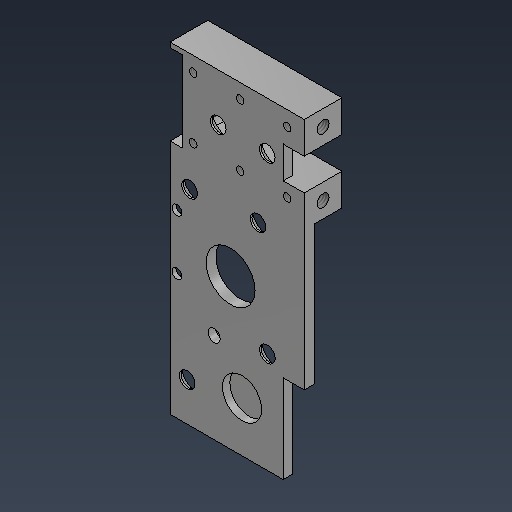
# Autodesk Inventor part: LeftGearboxCoverr
Saved by Autodesk Inventor 2026.2 (Build 302298010, 298A)
## iProperties
Created: 2026-04-13
Part Number: LeftGearboxCoverr
Material: Nylon 6/6
Document SubType Name: Modeling
Designer: szymo
Density: 1.13 g/cm^3
Appearance: Nylon 6(1)
Mass: 4.78265 g
Surface Area: 44.1112 cm^2
Volume: 4.23243 cm^3
Author: szymo
Autodesk Inventor part; units mm, degrees
ref_plane "YZ Plane" through (0, 0, 0) normal (1, 0, 0) x (0, 1, 0)
ref_plane "XZ Plane" through (0, 0, 0) normal (0, 1, 0) x (-1, 0, 0)
ref_plane "XY Plane" through (0, 0, 0) normal (0, 0, 1) x (1, 0, 0)
sketch "Sketch1" plane through (0, 0, 0) normal (0, 0, 1) x (1, 0, 0)
  circle A0 centre (14.7, -55.6371) radius 14.7 construction
  circle A1 centre (12.35, -35.2722) radius 5
  circle A2 centre (14.7, -14.7) radius 14.7 construction
  line L0 (23.1, -65.8371) -> (0, -65.8371)
  line L1 (0, -65.8371) -> (0, 0)
  line L2 (0, 0) -> (27.4, 0)
  line L3 (27.4, 0) -> (27.4, -19.5)
  line L4 (2.5, -1) -> (2.5, -9.4261)
  line L5 (2.5, -1) -> (1, -1)
  line L6 (1, -1) -> (1, -1)
  line L7 (1, -1) -> (0, -1)
  line L8 (2.5, -9.4261) -> (2.5, -17.5)
  line L9 (2.5, -17.5) -> (1, -17.5)
  line L10 (1, -17.5) -> (1, -17.5)
  line L11 (1, -17.5) -> (0, -17.5)
  line L12 (7.8075, -6.5) -> (27.4, -6.5)
  line L13 (7.8075, -6.5) -> (2.5, -6.5)
  line L14 (2.5, -13) -> (27.4, -13)
  line L15 (0, -19.5) -> (27.4, -19.5)
  circle A3 centre (14.7, -55.6371) radius 4
  circle A4 centre (9.002, -47.4193) radius 1.25
  line L16 (23.1, -13) -> (23.1, -6.5)
  circle A5 centre (14.7, -55.6371) radius 14.7 projected
  circle A6 centre (14.7, -55.6371) radius 14 projected
  line L17 (6.8877, -8.4575) -> (4.7029, -7.1961) projected
  arc A7 (4.7029, -7.1961) -> (3.2029, -9.7942) centre (14.7, -14.7) ccw projected
  line L18 (3.2029, -9.7942) -> (5.3877, -11.0556) projected
  arc A8 (6.8877, -8.4575) -> (5.3877, -11.0556) centre (14.7, -14.7) ccw projected
  arc A9 (24.6971, -22.2039) -> (26.1971, -19.6058) centre (14.7, -14.7) ccw projected
  line L19 (26.1971, -19.6058) -> (24.0123, -18.3444) projected
  arc A10 (22.5123, -20.9425) -> (24.0123, -18.3444) centre (14.7, -14.7) ccw projected
  line L20 (22.5123, -20.9425) -> (24.6971, -22.2039) projected
  circle A11 centre (14.7, -14.7) radius 5 projected
  circle A12 centre (14.7, -14.7) radius 14 projected
  circle A13 centre (14.7, -14.7) radius 14.7 projected
  circle A14 centre (14.7, -14.7) radius 14 projected
  circle A15 centre (12.35, -35.2722) radius 5 projected
  circle A16 centre (12.35, -35.2722) radius 5.4 projected
  line L21 (1.5, -1) -> (1.5, -17) projected
  line L22 (2.5, -1) -> (1.5, -1) projected
  line L23 (2.5, -17) -> (2.5, -1) projected
  line L24 (2.5, -17) -> (1.5, -17) projected
  circle A17 centre (9.002, -47.4193) radius 1.25 projected
  arc A18 (10.0798, -44.7809) -> (10.0692, -43.3571) centre (6.4391, -44.096) ccw projected
  arc A19 (10.4149, -44.9442) -> (10.0798, -44.7809) centre (9.002, -47.4193) ccw projected
  arc A20 (11.5425, -44.0747) -> (10.4149, -44.9442) centre (13.1986, -47.3885) ccw projected
  arc A21 (11.9573, -44.4349) -> (11.5425, -44.0747) centre (9.002, -47.4193) ccw projected
  arc A22 (11.2545, -45.6733) -> (11.9573, -44.4349) centre (8.4441, -43.2598) ccw projected
  arc A23 (11.4632, -45.9822) -> (11.2545, -45.6733) centre (9.002, -47.4193) ccw projected
  arc A24 (12.8744, -45.7931) -> (11.4632, -45.9822) centre (12.6518, -49.4909) ccw projected
  arc A25 (13.0535, -46.3124) -> (12.8744, -45.7931) centre (9.002, -47.4193) ccw projected
  arc A26 (11.8257, -47.0335) -> (13.0535, -46.3124) centre (10.5986, -43.5381) ccw projected
  arc A27 (11.8519, -47.4053) -> (11.8257, -47.0335) centre (9.002, -47.4193) ccw projected
  arc A28 (13.1687, -47.9471) -> (11.8519, -47.4053) centre (11.1269, -51.0383) ccw projected
  arc A29 (13.0641, -48.4865) -> (13.1687, -47.9471) centre (9.002, -47.4193) ccw projected
  arc A30 (11.6403, -48.497) -> (13.0641, -48.4865) centre (12.3253, -44.8564) ccw projected
  arc A31 (11.4771, -48.8322) -> (11.6403, -48.497) centre (9.002, -47.4193) ccw projected
  arc A32 (12.3465, -49.9598) -> (11.4771, -48.8322) centre (9.0327, -51.6159) ccw projected
  arc A33 (11.9863, -50.3746) -> (12.3465, -49.9598) centre (9.002, -47.4193) ccw projected
  arc A34 (10.748, -49.6718) -> (11.9863, -50.3746) centre (13.1615, -46.8614) ccw projected
  arc A35 (10.439, -49.8804) -> (10.748, -49.6718) centre (9.002, -47.4193) ccw projected
  arc A36 (10.6282, -51.2917) -> (10.439, -49.8804) centre (6.9303, -51.069) ccw projected
  arc A37 (10.1088, -51.4708) -> (10.6282, -51.2917) centre (9.002, -47.4193) ccw projected
  arc A38 (9.3878, -50.243) -> (10.1088, -51.4708) centre (12.8832, -49.0159) ccw projected
  arc A39 (9.0159, -50.2692) -> (9.3878, -50.243) centre (9.002, -47.4193) ccw projected
  arc A40 (8.4741, -51.586) -> (9.0159, -50.2692) centre (5.383, -49.5442) ccw projected
  arc A41 (7.9347, -51.4814) -> (8.4741, -51.586) centre (9.002, -47.4193) ccw projected
  arc A42 (7.9242, -50.0576) -> (7.9347, -51.4814) centre (11.5649, -50.7425) ccw projected
  arc A43 (7.589, -49.8944) -> (7.9242, -50.0576) centre (9.002, -47.4193) ccw projected
  arc A44 (6.4615, -50.7638) -> (7.589, -49.8944) centre (4.8053, -47.45) ccw projected
  arc A45 (6.0467, -50.4036) -> (6.4615, -50.7638) centre (9.002, -47.4193) ccw projected
  arc A46 (6.7494, -49.1652) -> (6.0467, -50.4036) centre (9.5599, -51.5788) ccw projected
  arc A47 (6.5408, -48.8563) -> (6.7494, -49.1652) centre (9.002, -47.4193) ccw projected
  arc A48 (5.1296, -49.0454) -> (6.5408, -48.8563) centre (5.3522, -45.3476) ccw projected
  arc A49 (4.9504, -48.5261) -> (5.1296, -49.0454) centre (9.002, -47.4193) ccw projected
  arc A50 (6.1782, -47.805) -> (4.9504, -48.5261) centre (7.4054, -51.3004) ccw projected
  arc A51 (6.152, -47.4332) -> (6.1782, -47.805) centre (9.002, -47.4193) ccw projected
  arc A52 (4.8353, -46.8914) -> (6.152, -47.4332) centre (6.877, -43.8003) ccw projected
  arc A53 (4.9398, -46.352) -> (4.8353, -46.8914) centre (9.002, -47.4193) ccw projected
  arc A54 (6.3636, -46.3415) -> (4.9398, -46.352) centre (5.6787, -49.9822) ccw projected
  arc A55 (6.5269, -46.0063) -> (6.3636, -46.3415) centre (9.002, -47.4193) ccw projected
  arc A56 (5.6574, -44.8788) -> (6.5269, -46.0063) centre (8.9712, -43.2226) ccw projected
  arc A57 (6.0177, -44.4639) -> (5.6574, -44.8788) centre (9.002, -47.4193) ccw projected
  arc A58 (7.256, -45.1667) -> (6.0177, -44.4639) centre (4.8425, -47.9771) ccw projected
  arc A59 (7.5649, -44.9581) -> (7.256, -45.1667) centre (9.002, -47.4193) ccw projected
  arc A60 (7.3758, -43.5469) -> (7.5649, -44.9581) centre (11.0736, -43.7695) ccw projected
  arc A61 (7.8951, -43.3677) -> (7.3758, -43.5469) centre (9.002, -47.4193) ccw projected
  arc A62 (8.6162, -44.5955) -> (7.8951, -43.3677) centre (5.1208, -45.8227) ccw projected
  arc A63 (8.9881, -44.5693) -> (8.6162, -44.5955) centre (9.002, -47.4193) ccw projected
  arc A64 (9.5298, -43.2526) -> (8.9881, -44.5693) centre (12.621, -45.2943) ccw projected
  arc A65 (10.0692, -43.3571) -> (9.5298, -43.2526) centre (9.002, -47.4193) ccw projected
  circle A66 centre (23.925, -15.5491) radius 0.75
  circle A67 centre (4.725, -15.5491) radius 0.75
  circle A68 centre (14.325, -3) radius 0.75
  line L25 (23.1, -19.5) -> (23.1, -65.8371)
  circle A69 centre (12.35, -35.2722) radius 15
  line L26 (23.1, -47.8371) -> (27.4, -47.8371)
  line L27 (27.4, -47.8371) -> (27.4, -19.5)
  line L28 (23.1, -9.3) -> (2.5, -9.3)
  circle A70 centre (23.925, -3.0509) radius 0.75
  circle A71 centre (4.725, -3.0509) radius 0.75
  circle A72 centre (14.325, -15.6) radius 0.75
  point P0 (2.5, -13)
  point P1 (5.6825, -44.928)
  point P2 (6.1849, -44.5244)
  point P3 (7.3696, -43.7096)
  point P4 (7.9154, -43.3909)
  point P5 (0.2691, -17.5)
  point P6 (0, -14.7)
  dimension "d23" = 8
  dimension "d26" = 2.5
  dimension "d32" = 19.5
  dimension "d33" = 6.5
  dimension "d34" = 0.5
  dimension "d35" = 0.5
  dimension "d36" = 0
  dimension "d37" = 0
  dimension "d42" = 4.5
  dimension "d43" = 6.5
  dimension "d58" = 2
  dimension "d59" = 6.3
  dimension "d79" = 30
  dimension "d80" = 18
  dimension "d81" = 3.15
  constraints: 42 end point, 13 point on line, 12 centre point, 12 coincident, 12 perpendicular, 6 symmetric about line, 5 horizontal, 5 tangent, 3 parallel, 2 collinear, 1 vertical, 14 other
  measures "d23" diameter of A3
  measures "d26" diameter of A4
  measures "d32" distance between parallel lines of L15 L2
  measures "d33" distance between parallel lines of L15 L14
  measures "d34" distance between parallel lines of L9 L24
  measures "d35" distance between parallel lines of L10 L21
  measures "d36" distance between parallel lines of L11 L9
  measures "d37" distance between parallel lines of L7 L5
  measures "d42" distance edge to line of A0 L0
  measures "d43" distance between parallel lines of L12 L2
  measures "d58" distance edge to line of A2 L3
  measures "d59" distance edge to line of A2 L25
  measures "d79" diameter of A69
  measures "d80" distance between parallel lines of L0 L26
  measures "d81" distance edge to line of A72 L15
extrude "Extrusion3" add sketch "Sketch1" against normal blind 2 contours L0 A6 A69 A50 A49 A48 A46 A45 A44 A43 A42 A41 A40 A39 A38 A37 A36 A34 A33 L25 | L0 A5 A69 A6 | L25 A69 A6 L26 | L0 L1 A5 | A69 A5 L25 A6 A62 A61 A60 A58 A57 A56 | A6 A56 A55 A54 A53 A52 A51 A50 A69 | A69 A33 A32 A31 A30 A29 A28 A27 A26 A25 A24 A23 A22 A21 A20 A19 A18 A65 A64 A63 A62 A6 L25 | L25 A6 A69 | A6 A69 A5 L26 | L1 A69 A5 | A56 A57 A58 A6 | A6 A58 A59 A60 A62 A63 A64 A65 A18 A19 A20 A21 A22 A23 A24 A25 A26 A27 A28 A29 A30 A31 A32 A33 A69 A34 A35 A36 A46 A47 A48 A50 A51 A52 A53 A54 A55 A56 | A69 L1 A13 L25 A5 | A69 A48 A49 A50 | L25 A5 A69 A6 | A33 A34 A69 | A5 A69 A13 L27 L26 | A6 A60 A59 A58 | L25 A13 A69 A5 | A48 A47 A46 A69 | A6 A60 A61 A62 | A69 A36 A35 A34 | L1 L15 A13 A69 | L25 A12 A69 A13 | A13 A69 A12 L25 | A69 A36 A37 A38 A39 A40 A41 A42 A43 A44 A45 A46 | A13 A69 A12 L27 | L1 L11 A13 L15 | A13 L15 A12 A69 | L25 A69 A12 | A12 A69 L25 | A12 A69 L25 L20 A9 L19 L15 L27 | A13 L11 A12 L15 | A12 L15 A11 L25 A10 L20 A69 | L15 L19 A10 A11 L14 L3 | A12 L11 L9 L8 L14 A11 L15 | L25 A10 L15 L19 A9 L20 | L20 A10 L25 | L12 A13 A70 L2 L3 | L12 A12 L13 A13 A71 A70 | L15 A10 L19 | L1 L2 A13 A71 L4 L5 L7 | A11 L14 L15 | L15 A11 | L25 L15 A10 | L12 L13 A12 | A70 A13 | A13 A70 | L14 A11 L8 L4 L28 A7 L18 A8 L16 | L13 A12 L4 | A11 L14 | L16 L28 A8 L17 A7 L4 A12 L13 L12 | A71 A13 | A13 A71 | L28 A7 L17 A8 | A8 L18 A7 L28 | A3 | A4 | A16 | A66 | A67 | A68 | A72
ref_plane "Work Plane1" through (1, -19, -6.7) normal (0, 0, 1) x (1, 0, 0)
ref_plane "Work Plane2" through (1, -19, -7.7) normal (0, 0, 1) x (1, 0, 0)
extrude "Extrusion4" add sketch "Sketch1" against normal up to surface (7.7 mm away) contours L1 L11 A13 L15 | A13 L11 A12 L15 | L15 L19 A10 A11 L14 L3 | A12 L11 L9 L8 L14 A11 L15 | L12 A13 A70 L2 L3 | L12 A12 L13 A13 A71 A70 | L15 A10 L19 | L1 L2 A13 A71 L4 L5 L7 | A11 L14 L15 | L12 L13 A12 | A70 A13 | A13 A70 | A71 A13 | A13 A71 | A66 | A67 | A68 | A72
hole "Hole1" at (23.925, -15.5491, 0) at (4.725, -15.5491, 0) at (14.325, -3, 0) at (14.325, -15.6, 0) at (4.725, -3.0509, 0) at (23.925, -3.0509, 0) direction (0, 0, -1) diameter 1.567 end through all thread size "M2x0.4" class "6H" standard "ISO Metric profile"
extrude "Extrusion5" cut sketch "Sketch1" against normal blind 1.5 contours A3 | A4
sketch "Sketch2" plane through (0, 0, -2) normal (0, 0, -1) x (-1, 0, 0)
  line L0 (-2.5, -17.5) -> (0, -17.5) projected
  line L1 (-2.5, -1) -> (-2.5, -17.5) projected
  line L2 (0, -1) -> (-2.5, -1) projected
  line L3 (0, -17.5) -> (0, -65.8371) projected
  line L4 (-27.4, 0) -> (0, 0) projected
  line L5 (-27.4, -6.5) -> (-27.4, 0) projected
  line L6 (-23.1, -6.5) -> (-27.4, -6.5) projected
  line L7 (-23.1, -65.8371) -> (-23.1, -6.5) projected
  line L8 (0, -65.8371) -> (-23.1, -65.8371) projected
  line L9 (0, 0) -> (0, -1) projected
  arc A0 (-16.7767, -44.2391) -> (-16.5957, -51.0104) centre (-9.002, -47.4193) ccw projected
  arc A1 (-3.9544, -40.7049) -> (-16.7767, -44.2391) centre (-12.35, -35.2722) ccw projected
  circle A2 centre (-9.0431, -61.2939) radius 2.25 projected
  circle A3 centre (-1.4, -29.0252) radius 0.7 projected
  circle A4 centre (-1.4, -40.2691) radius 0.7 projected
  arc A5 (-9.7023, -55.79) -> (-3.9544, -40.7049) centre (-9.002, -47.4193) ccw projected
  circle A6 centre (-17.9752, -23) radius 1.2295 projected
  circle A7 centre (-9.85, -9.75) radius 1.2295 projected
  circle A8 centre (-19.85, -9.75) radius 1.2295 projected
  circle A9 centre (-19.873, -45.2549) radius 1.2295 projected
  circle A10 centre (-4, -24.0349) radius 1.2295 projected
  circle A11 centre (-3.5, -57.971) radius 1.2295 projected
  circle A12 centre (-20.3569, -49.9802) radius 2.25 projected
  circle A13 centre (-20.3569, -49.9802) radius 2.25 projected
  arc A14 (-16.5957, -51.0104) -> (-9.7023, -55.79) centre (-14.7, -55.6371) ccw projected
  point P0 (-19.873, -45.2549)
  point P1 (-3.5, -57.971)
  point P2 (-4, -24.0349)
  point P3 (-17.9752, -23)
  point P4 (-19.85, -9.75)
  point P5 (-9.85, -9.75)
  point P6 (-19.873, -45.2549)
  point P7 (-20.3569, -49.9802)
  point P8 (-19.873, -45.2549)
  point P9 (-19.873, -45.2549)
  point P10 (-9.002, -47.4193)
  point P11 (-12.35, -35.2722)
  point P12 (-14.7, -55.6371)
  point P13 (-12.35, -35.2722)
  point P14 (-14.7, -55.6371)
  point P15 (-12.35, -35.2722)
  point P16 (-14.7, -55.6371)
  point P17 (-19.873, -45.2549)
  point P18 (-9.002, -47.4193)
  point P19 (-14.7, -55.6371)
  point P20 (-19.873, -45.2549)
  point P21 (-21.2554, -47.9174)
  point P22 (-12.35, -35.2722)
  point P23 (-14.7, -55.6371)
  point P24 (-19.0589, -48.1424)
  point P25 (-19.873, -45.2549)
  point P26 (-14.7, -55.6371)
  point P27 (-20.3569, -49.9802)
  point P28 (-19.873, -45.2549)
  point P29 (-12.35, -35.2722)
  point P30 (-19.873, -45.2549)
  point P31 (-14.7, -55.6371)
  point P32 (-20.3569, -49.9802)
  point P33 (-19.873, -45.2549)
  point P34 (-12.35, -35.2722)
  point P35 (-19.873, -45.2549)
  point P36 (-14.7, -55.6371)
  point P37 (-20.3569, -49.9802)
  point P38 (-19.873, -45.2549)
  point P39 (-12.35, -35.2722)
  point P40 (-19.873, -45.2549)
  point P41 (-14.7, -55.6371)
  point P42 (-20.3569, -49.9802)
  point P43 (-19.873, -45.2549)
  point P44 (-12.35, -35.2722)
  point P45 (-19.873, -45.2549)
  point P46 (-14.7, -55.6371)
  point P47 (-20.3569, -49.9802)
  point P48 (-19.873, -45.2549)
  point P49 (-12.35, -35.2722)
  point P50 (-19.873, -45.2549)
  point P51 (-20.3569, -49.9802)
  point P52 (-9.002, -47.4193)
  point P53 (-12.35, -35.2722)
  point P54 (-9.002, -47.4193)
  point P55 (-9.002, -47.4193)
  point P56 (-9.002, -47.4193)
  point P57 (-9.002, -47.4193)
  point P58 (-9.002, -47.4193)
  point P59 (-9.002, -47.4193)
  point P60 (-9.002, -47.4193)
  point P61 (-9.002, -47.4193)
  point P62 (-9.002, -47.4193)
  point P63 (-9.002, -47.4193)
  point P64 (-9.002, -47.4193)
  point P65 (-9.002, -47.4193)
  point P66 (-9.002, -47.4193)
  point P67 (-9.002, -47.4193)
  point P68 (-9.002, -47.4193)
  point P69 (-9.002, -47.4193)
  point P70 (-9.002, -47.4193)
  point P71 (-9.002, -47.4193)
  point P72 (-9.002, -47.4193)
  point P73 (-9.002, -47.4193)
  point P74 (-9.002, -47.4193)
  point P75 (-9.002, -47.4193)
  point P76 (-9.002, -47.4193)
  point P77 (-9.002, -47.4193)
  point P78 (-9.002, -47.4193)
  point P79 (-9.002, -47.4193)
hole "Hole2" at (19.873, -45.2549, -2) at (3.5, -57.971, -2) at (4, -24.0349, -2) at (17.9752, -23, -2) at (19.85, -9.75, -2) at (9.85, -9.75, -2) direction (0, 0, 1) diameter 3.2 depth 5 countersink diameter 6.5 countersink angle 90 clearance for "Countersunk Flat Head Screw ISO 2009/7046" size "M3" standard "ISO"
sketch "Sketch3" plane through (27.4, -6.5, 0) normal (1, 0, 0) x (0, 0, -1)
  line L0 (0, 0) -> (0, 6.5) projected
  line L1 (7.7, 6.5) -> (7.7, 0) projected
  line L2 (0, 6.5) -> (7.7, 6.5) projected
  line L3 (0, -6.5) -> (0, 0) projected
  line L4 (0, 0) -> (7.7, 6.5)
  line L5 (0, 6.5) -> (7.7, 0)
  line L6 (0, 0) -> (7.7, 0) projected
  line L7 (0, -13) -> (7.7, -6.5)
  line L8 (7.7, -13) -> (0, -6.5)
  point P0 (0, 6.5)
  point P1 (3.85, 3.25)
  point P2 (3.85, -9.75)
  constraints: 8 end point, 2 midpoint
hole "Hole3" at (27.4, -3.25, -3.85) at (27.4, -16.25, -3.85) direction (-1, 0, 0) diameter 2.459 depth 10 thread size "M3x0.5" class "6H" standard "ISO Metric profile"
sketch "Sketch4" plane through (0, 0, -2) normal (0, 0, -1) x (-1, 0, 0)
  circle A0 centre (-1.4, -40.2691) radius 0.7 projected
  circle A1 centre (-1.4, -29.0252) radius 0.7 projected
  circle A2 centre (-1.4, -40.2691) radius 2
  circle A3 centre (-1.4, -29.0252) radius 2
  line L0 (-1.4, -42.2691) -> (0.6, -42.2691)
  line L1 (0.6, -42.2691) -> (0.6, -38.2691)
  line L2 (0.6, -38.2691) -> (-1.4, -38.2691)
  line L3 (-1.4, -38.2691) -> (-1.4, -42.2691)
  line L4 (-1.4, -27.0252) -> (0.6, -27.0252)
  line L5 (0.6, -27.0252) -> (0.6, -31.0252)
  line L6 (0.6, -31.0252) -> (-1.4, -31.0252)
  line L7 (-1.4, -31.0252) -> (-1.4, -27.0252)
  point P0 (0, 0)
  point P1 (-1.4, -31.0252)
  point P2 (-1.4, -38.2691)
  dimension "d60" = 4
  dimension "d61" = 4
  constraints: 16 end point, 5 horizontal, 4 parallel, 2 coincident, 2 perpendicular, 2 vertical, 1 point on line, 6 other
extrude "Extrusion7" cut sketch "Sketch4" against normal blind 1.2
sketch "Sketch5" plane through (0, 0, -2) normal (0, 0, -1) x (-1, 0, 0)
  arc A0 (-1.4, -38.2691) -> (-1.4, -42.2691) centre (-1.4, -40.2691) ccw projected
  arc A1 (-1.4, -27.0252) -> (-1.4, -31.0252) centre (-1.4, -29.0252) ccw projected
  point P0 (0, 0)
hole "Hole4" at (1.4, -40.2691, -2) at (1.4, -29.0252, -2) direction (0, 0, 1) diameter 2 end through all clearance for "Countersunk Flat Head Screw ISO 2009/7046" size "M2" standard "ISO"
chamfer "Chamfer2" distance 2 angle 25 2 edges at (2.5, -6.5, -4.85) (2.5, -13, -4.85) measured on face at (2.5, -13.5, -4.85) measured on face at (2.5, -6, -4.85)
fillet "Fillet1" radius 4 4 edges at (2.5, -15, -4.85) (3.4326, -13, -4.85) (3.4326, -6.5, -4.85) (2.5, -4.5, -4.85)
body "Solid3"
